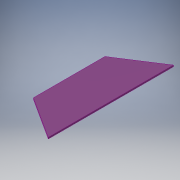
# Autodesk Inventor part: Top + Spinner
Saved by Autodesk Inventor 2017 (Build 210142000, 142)
## iProperties
Created: 2017-06-10
Part Number: Top + Spinner
Material: Generic
Document SubType Name: Modeling
Designer: Matthew
Density: 1 g/cm^3
Appearance: Smooth - Purple
Author: Matthew
Autodesk Inventor part; units mm, degrees
ref_plane "YZ Plane" through (0, 0, 0) normal (1, 0, 0) x (0, 1, 0)
ref_plane "XZ Plane" through (0, 0, 0) normal (0, 1, 0) x (-1, 0, 0)
ref_plane "XY Plane" through (0, 0, 0) normal (0, 0, 1) x (1, 0, 0)
sketch "Sketch1" plane through (0, 0, 0) normal (0, 1, 0) x (-1, 0, 0)
  line L0 (88.9, -57.15) -> (88.9, -209.55)
  line L1 (88.9, -209.55) -> (0, -266.7)
  line L2 (0, -266.7) -> (0, 0)
  line L3 (0, 0) -> (88.9, -57.15)
  dimension "d0" = 152.4
  dimension "d1" = 88.9
  dimension "d2" = 266.7
  constraints: 8 end point, 1 equal length, 1 parallel, 1 vertical
  measures "d0" distance of L0.start L0.end
  measures "d1" distance between parallel lines of L2 L0
  measures "d2" distance of L1.end L2.end
extrude "Extrusion1" add sketch "Sketch1" along normal blind 3.175
ref_plane "Work Plane1" through (0, 0, 0) normal (0, 0, -1) x (0, 1, 0)
body "Solid1"
